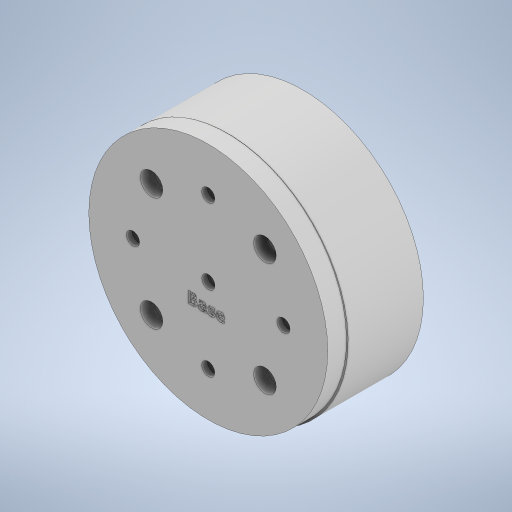
# Autodesk Inventor part: adaptor_spine_base_names
Saved by Autodesk Inventor 2024 (Build 280153000, 153)
## iProperties
Created: 2024-05-24
Part Number: adaptor_spine_base_names
Material: Generic
Document SubType Name: Modeling
Designer: maint
Density: 1 g/cm^3
Appearance: Default
Author: maint
Autodesk Inventor part; units mm, degrees
ref_plane "YZ Plane" through (0, 0, 0) normal (1, 0, 0) x (0, 1, 0)
ref_plane "XZ Plane" through (0, 0, 0) normal (0, 1, 0) x (-1, 0, 0)
ref_plane "XY Plane" through (0, 0, 0) normal (0, 0, 1) x (1, 0, 0)
sketch "Sketch1" plane through (0, 0, 0) normal (0, 0, 1) x (1, 0, 0)
  line L0 (40, -40) -> (-40, -40)
  line L1 (-40, -40) -> (-40, 40)
  line L2 (-40, 40) -> (40, 40)
  line L3 (40, 40) -> (40, -40)
  line L4 (40, -40) -> (-40, 40) construction
  line L5 (-40, -40) -> (40, 40) construction
  circle A0 centre (0, 0) radius 63.5
  dimension "d0" = 80
  dimension "d72" = 127
  constraints: 12 end point, 2 midpoint, 2 parallel, 2 perpendicular, 1 centre point, 1 coincident, 1 horizontal
  measures "d0" distance of L1.end L2.end
  measures "d72" diameter of A0
extrude "Extrusion1" add sketch "Sketch1" along normal blind 10 contours L0 L1 L2 L3 | A0
sketch "Sketch2" plane through (0, 0, 0) normal (0, 0, -1) x (-1, 0, 0)
  arc A0 (40, 37) -> (37, 40) centre (37, 37) ccw
  line L0 (30.15, -30.15) -> (-30.15, -30.15)
  line L1 (-30.15, -30.15) -> (-30.15, 30.15)
  line L2 (-30.15, 30.15) -> (30.15, 30.15)
  line L3 (30.15, 30.15) -> (30.15, -30.15)
  line L4 (30.15, -30.15) -> (-30.15, 30.15) construction
  line L5 (-30.15, -30.15) -> (30.15, 30.15) construction
  circle A1 centre (-30.15, 30.15) radius 4.75
  circle A2 centre (30.15, 30.15) radius 4.75
  circle A3 centre (30.15, -30.15) radius 4.75
  circle A4 centre (-30.15, -30.15) radius 4.75
  point P0 (0, 0)
  point P1 (39.1213, 39.1213)
  dimension "d32" = 60.3
  dimension "d33" = 9.5
  constraints: 12 end point, 5 centre point, 4 coincident, 3 equal radius, 3 point on circle, 2 midpoint, 2 parallel, 2 perpendicular, 1 horizontal
  measures "d32" distance of L1.end L2.end
  measures "d33" diameter of A2
hole "Hole3" at (30.15, -30.15, 0) at (30.15, 30.15, 0) at (-30.15, 30.15, 0) at (-30.15, -30.15, 0) direction (0, 0, 1) diameter 6.6 end through all
sketch "Sketch3" plane through (0, 0, 0) normal (0, 0, -1) x (-1, 0, 0)
  circle A0 centre (0, 0) radius 40
  circle A1 centre (0, 40) radius 2.5
  circle A2 centre (40, 0) radius 2.5
  circle A3 centre (0, -40) radius 2.5
  circle A4 centre (-40, 0) radius 2.5
  circle A5 centre (-0.0779, 0.0489) radius 2.5
  dimension "d12" = 5
  dimension "d60" = 80
  dimension "d74" = 5
  constraints: 6 centre point, 4 point on circle, 3 equal radius
  measures "d12" diameter of A1
  measures "d60" diameter of A0
  measures "d74" diameter of A5
hole "Hole1" at (40, 0, 0) at (0, 40, 0) at (0, -40, 0) at (-40, 0, 0) at (0.0779, 0.0489, 0) direction (0, 0, 1) diameter 7 end through all
sketch "Sketch8" plane through (0, 0, 0) normal (0, 0, -1) x (-1, 0, 0)
  circle A0 centre (0, 0) radius 40
  circle A1 centre (0, 40) radius 12.0233
  circle A2 centre (40, 0) radius 12.001
  circle A3 centre (-40, 0) radius 12.185
  circle A4 centre (0, -40) radius 12.001
  circle A5 centre (-0.3746, -0.3656) radius 12.0233
  dimension "d61" = 80
  constraints: 6 centre point, 4 point on circle
  measures "d61" diameter of A0
hole "Hole4" at (-40, 0, 0) at (0, 40, 0) at (40, 0, 0) at (0, -40, 0) at (0.3746, -0.3656, 0) direction (0, 0, 1) diameter 17 depth 7
sketch "Sketch10" plane through (0, 0, 10) normal (0, 0, 1) x (1, 0, 0)
  circle A0 centre (30.15, 30.15) radius 3.3 projected
  circle A1 centre (30.15, 30.15) radius 6
  circle A2 centre (-30.15, 30.15) radius 3.3 projected
  circle A3 centre (-30.15, 30.15) radius 6
  circle A4 centre (-30.15, -30.2444) radius 6
  circle A5 centre (30.15, -30.2444) radius 6
  point P0 (0, 0)
  dimension "d63" = 12
  constraints: 4 centre point, 3 equal radius, 2 coincident
  measures "d63" diameter of A1
hole "Hole5" at (-30.15, -30.2444, 10) at (30.15, -30.2444, 10) at (30.15, 30.15, 10) at (-30.15, 30.15, 10) direction (0, 0, -1) diameter 12 depth 7
sketch "Sketch11" plane through (-1.9817, 2.6504, 0) normal (0, 0, -1) x (-1, 0, 0)
  line L0 (-12.9782, -14.2221) -> (9.0418, -14.2221) construction
  line L1 (9.0418, -14.2221) -> (9.0418, -6.8756) construction
  line L2 (9.0418, -6.8756) -> (-12.9782, -6.8756) construction
  line L3 (-12.9782, -6.8756) -> (-12.9782, -14.2221) construction
  spline S0 degree 2 poles (-10.4621, -20.5396) (-11.164, -20.5396) (-12.2219, -20.2677) (-12.6767, -20.07) knots 0 0 0 1 2 2 2
  line L4 (-12.6767, -20.07) -> (-12.6767, -18.6166)
  line L5 (-12.6767, -18.6166) -> (-12.5383, -18.6166)
  spline S1 degree 2 poles (-12.5383, -18.6166) (-12.0785, -19.0072) (-10.9762, -19.4273) (-10.4571, -19.4273) knots 0 0 0 1 2 2 2
  spline S2 degree 2 poles (-10.4571, -19.4273) (-10.3237, -19.4273) (-9.8936, -19.368) (-9.7651, -19.3087) knots 0 0 0 1 2 2 2
  spline S3 degree 2 poles (-9.7651, -19.3087) (-9.6069, -19.2395) (-9.3845, -18.9874) (-9.3845, -18.7847) knots 0 0 0 1 2 2 2
  spline S4 degree 2 poles (-9.3845, -18.7847) (-9.3845, -18.5524) (-9.7453, -18.2657) (-9.9925, -18.2014) knots 0 0 0 1 2 2 2
  spline S5 degree 2 poles (-9.9925, -18.2014) (-10.3039, -18.1174) (-11.0108, -17.974) (-11.3222, -17.8653) knots 0 0 0 1 2 2 2
  spline S6 degree 2 poles (-11.3222, -17.8653) (-12.0291, -17.6181) (-12.6421, -16.7728) (-12.6421, -16.1401) knots 0 0 0 1 2 2 2
  spline S7 degree 2 poles (-12.6421, -16.1401) (-12.6421, -15.2849) (-11.1937, -14.2221) (-10.1062, -14.2221) knots 0 0 0 1 2 2 2
  spline S8 degree 2 poles (-10.1062, -14.2221) (-9.5624, -14.2221) (-8.4848, -14.4445) (-8.0597, -14.6324) knots 0 0 0 1 2 2 2
  line L6 (-8.0597, -14.6324) -> (-8.0597, -16.0264)
  line L7 (-8.0597, -16.0264) -> (-8.1931, -16.0264)
  spline S9 degree 2 poles (-8.1931, -16.0264) (-8.5342, -15.7347) (-9.513, -15.3343) (-10.0271, -15.3343) knots 0 0 0 1 2 2 2
  spline S10 degree 2 poles (-10.0271, -15.3343) (-10.2298, -15.3343) (-10.5461, -15.3936) (-10.7241, -15.4727) knots 0 0 0 1 2 2 2
  spline S11 degree 2 poles (-10.7241, -15.4727) (-10.8674, -15.537) (-11.0751, -15.794) (-11.0751, -15.9522) knots 0 0 0 1 2 2 2
  spline S12 degree 2 poles (-11.0751, -15.9522) (-11.0751, -16.1895) (-10.7439, -16.4614) (-10.2693, -16.5701) knots 0 0 0 1 2 2 2
  spline S13 degree 2 poles (-10.2693, -16.5701) (-9.9628, -16.6393) (-9.3943, -16.7728) (-9.0681, -16.8865) knots 0 0 0 1 2 2 2
  spline S14 degree 2 poles (-9.0681, -16.8865) (-8.4353, -17.1188) (-7.8174, -17.89) (-7.8174, -18.5227) knots 0 0 0 1 2 2 2
  spline S15 degree 2 poles (-7.8174, -18.5227) (-7.8174, -19.4323) (-9.246, -20.5396) (-10.4621, -20.5396) knots 0 0 0 1 2 2 2
  spline S16 degree 2 poles (-2.3403, -16.2538) (-2.3403, -16.6789) (-2.6122, -17.45) (-2.8643, -17.7071) knots 0 0 0 1 2 2 2
  spline S17 degree 2 poles (-2.8643, -17.7071) (-3.0175, -17.8702) (-3.3932, -18.1371) (-3.6157, -18.2311) knots 0 0 0 1 2 2 2
  spline S18 degree 2 poles (-3.6157, -18.2311) (-3.843, -18.325) (-4.372, -18.4337) (-4.6982, -18.4337) knots 0 0 0 1 2 2 2
  line L8 (-4.6982, -18.4337) -> (-5.499, -18.4337)
  line L9 (-5.499, -18.4337) -> (-5.499, -20.4308)
  line L10 (-5.499, -20.4308) -> (-7.0315, -20.4308)
  line L11 (-7.0315, -20.4308) -> (-7.0315, -14.3308)
  line L12 (-7.0315, -14.3308) -> (-4.6636, -14.3308)
  spline S19 degree 2 poles (-4.6636, -14.3308) (-4.1396, -14.3308) (-3.3734, -14.5236) (-3.062, -14.7312) knots 0 0 0 1 2 2 2
  spline S20 degree 2 poles (-3.062, -14.7312) (-2.716, -14.9636) (-2.3403, -15.7248) (-2.3403, -16.2538) knots 0 0 0 1 2 2 2
  spline S21 degree 2 poles (-3.9122, -16.2933) (-3.9122, -16.0313) (-4.1594, -15.6606) (-4.3275, -15.5914) knots 0 0 0 1 2 2 2
  spline S22 degree 2 poles (-4.3275, -15.5914) (-4.545, -15.4974) (-4.9404, -15.4678) (-5.2815, -15.4678) knots 0 0 0 1 2 2 2
  line L13 (-5.2815, -15.4678) -> (-5.499, -15.4678)
  line L14 (-5.499, -15.4678) -> (-5.499, -17.2968)
  line L15 (-5.499, -17.2968) -> (-5.3903, -17.2968)
  spline S23 degree 2 poles (-5.3903, -17.2968) (-5.1777, -17.2968) (-4.7922, -17.2869) (-4.6488, -17.2622) knots 0 0 0 1 2 2 2
  spline S24 degree 2 poles (-4.6488, -17.2622) (-4.5252, -17.2424) (-4.2533, -17.1238) (-4.1792, -17.0496) knots 0 0 0 1 2 2 2
  spline S25 degree 2 poles (-4.1792, -17.0496) (-4.021, -16.9013) (-3.9122, -16.5701) (-3.9122, -16.2933) knots 0 0 0 1 2 2 2
  line L16 (1.5155, -20.4308) -> (-1.7669, -20.4308)
  line L17 (-1.7669, -20.4308) -> (-1.7669, -19.368)
  line L18 (-1.7669, -19.368) -> (-0.8919, -19.368)
  line L19 (-0.8919, -19.368) -> (-0.8919, -15.3936)
  line L20 (-0.8919, -15.3936) -> (-1.7669, -15.3936)
  line L21 (-1.7669, -15.3936) -> (-1.7669, -14.3308)
  line L22 (-1.7669, -14.3308) -> (1.5155, -14.3308)
  line L23 (1.5155, -14.3308) -> (1.5155, -15.3936)
  line L24 (1.5155, -15.3936) -> (0.6405, -15.3936)
  line L25 (0.6405, -15.3936) -> (0.6405, -19.368)
  line L26 (0.6405, -19.368) -> (1.5155, -19.368)
  line L27 (1.5155, -19.368) -> (1.5155, -20.4308)
  line L28 (7.7588, -20.4308) -> (6.2857, -20.4308)
  line L29 (6.2857, -20.4308) -> (3.9327, -16.1796)
  line L30 (3.9327, -16.1796) -> (3.9327, -20.4308)
  line L31 (3.9327, -20.4308) -> (2.5338, -20.4308)
  line L32 (2.5338, -20.4308) -> (2.5338, -14.3308)
  line L33 (2.5338, -14.3308) -> (4.4122, -14.3308)
  line L34 (4.4122, -14.3308) -> (6.3599, -17.8257)
  line L35 (6.3599, -17.8257) -> (6.3599, -14.3308)
  line L36 (6.3599, -14.3308) -> (7.7588, -14.3308)
  line L37 (7.7588, -14.3308) -> (7.7588, -20.4308)
  line L38 (8.9996, -20.4308) -> (8.9996, -14.3308)
  line L39 (8.9996, -14.3308) -> (13.1223, -14.3308)
  line L40 (13.1223, -14.3308) -> (13.1223, -15.4925)
  line L41 (13.1223, -15.4925) -> (10.5221, -15.4925)
  line L42 (10.5221, -15.4925) -> (10.5221, -16.5652)
  line L43 (10.5221, -16.5652) -> (12.9196, -16.5652)
  line L44 (12.9196, -16.5652) -> (12.9196, -17.7268)
  line L45 (12.9196, -17.7268) -> (10.5221, -17.7268)
  line L46 (10.5221, -17.7268) -> (10.5221, -19.2692)
  line L47 (10.5221, -19.2692) -> (13.1223, -19.2692)
  line L48 (13.1223, -19.2692) -> (13.1223, -20.4308)
  line L49 (13.1223, -20.4308) -> (8.9996, -20.4308)
  point P0 (0, 0)
  constraints: 2 other
extrude "Extrusion5" cut sketch "Sketch11" against normal blind 1
sketch "Sketch12" plane through (-4.4722, 1.3995, 10) normal (0, 0, 1) x (1, 0, 0)
  line L0 (-6.7643, -10.3972) -> (19.0988, -10.3972) construction
  line L1 (19.0988, -10.3972) -> (19.0988, -6.1489) construction
  line L2 (19.0988, -6.1489) -> (-6.7643, -6.1489) construction
  line L3 (-6.7643, -6.1489) -> (-6.7643, -10.3972) construction
  spline S0 degree 2 poles (-1.2575, -14.6287) (-1.2575, -15.0834) (-1.6035, -15.7705) (-1.8902, -15.9979) knots 0 0 0 1 2 2 2
  spline S1 degree 2 poles (-1.8902, -15.9979) (-2.2362, -16.2698) (-3.0568, -16.4972) (-3.6945, -16.4972) knots 0 0 0 1 2 2 2
  line L4 (-3.6945, -16.4972) -> (-6.1315, -16.4972)
  line L5 (-6.1315, -16.4972) -> (-6.1315, -10.3972)
  line L6 (-6.1315, -10.3972) -> (-3.9812, -10.3972)
  spline S2 degree 2 poles (-3.9812, -10.3972) (-3.3089, -10.3972) (-2.6169, -10.501) (-2.3153, -10.6641) knots 0 0 0 1 2 2 2
  spline S3 degree 2 poles (-2.3153, -10.6641) (-1.9841, -10.8372) (-1.6628, -11.4304) (-1.6628, -11.8159) knots 0 0 0 1 2 2 2
  spline S4 degree 2 poles (-1.6628, -11.8159) (-1.6628, -12.2608) (-2.1077, -12.9578) (-2.5032, -13.121) knots 0 0 0 1 2 2 2
  line L7 (-2.5032, -13.121) -> (-2.5032, -13.1506)
  spline S5 degree 2 poles (-2.5032, -13.1506) (-1.9347, -13.2693) (-1.2575, -14.0058) (-1.2575, -14.6287) knots 0 0 0 1 2 2 2
  spline S6 degree 2 poles (-2.8393, -14.6039) (-2.8393, -14.3172) (-3.0667, -13.9959) (-3.2941, -13.9119) knots 0 0 0 1 2 2 2
  spline S7 degree 2 poles (-3.2941, -13.9119) (-3.4325, -13.8575) (-3.9219, -13.8476) (-4.3272, -13.8476) knots 0 0 0 1 2 2 2
  line L8 (-4.3272, -13.8476) -> (-4.609, -13.8476)
  line L9 (-4.609, -13.8476) -> (-4.609, -15.385)
  line L10 (-4.609, -15.385) -> (-4.525, -15.385)
  spline S8 degree 2 poles (-4.525, -15.385) (-3.9318, -15.385) (-3.477, -15.3701) (-3.2397, -15.2663) knots 0 0 0 1 2 2 2
  spline S9 degree 2 poles (-3.2397, -15.2663) (-3.0321, -15.1724) (-2.8393, -14.8264) (-2.8393, -14.6039) knots 0 0 0 1 2 2 2
  spline S10 degree 2 poles (-3.2199, -12.1175) (-3.2199, -11.9692) (-3.3732, -11.6577) (-3.5314, -11.5885) knots 0 0 0 1 2 2 2
  spline S11 degree 2 poles (-3.5314, -11.5885) (-3.6797, -11.5193) (-4.0949, -11.5094) (-4.5052, -11.5094) knots 0 0 0 1 2 2 2
  line L11 (-4.5052, -11.5094) -> (-4.609, -11.5094)
  line L12 (-4.609, -11.5094) -> (-4.609, -12.8046)
  line L13 (-4.609, -12.8046) -> (-4.4162, -12.8046)
  spline S12 degree 2 poles (-4.4162, -12.8046) (-4.0257, -12.8046) (-3.7093, -12.7898) (-3.5412, -12.7107) knots 0 0 0 1 2 2 2
  spline S13 degree 2 poles (-3.5412, -12.7107) (-3.3583, -12.6217) (-3.2199, -12.3201) (-3.2199, -12.1175) knots 0 0 0 1 2 2 2
  spline S14 degree 2 poles (2.0743, -16.0078) (1.926, -16.1314) (1.6937, -16.3291) (1.496, -16.428) knots 0 0 0 1 2 2 2
  spline S15 degree 2 poles (1.496, -16.428) (1.3032, -16.5219) (0.9374, -16.6208) (0.6111, -16.6208) knots 0 0 0 1 2 2 2
  spline S16 degree 2 poles (0.6111, -16.6208) (-0.0019, -16.6208) (-0.8076, -15.8002) (-0.8076, -15.1774) knots 0 0 0 1 2 2 2
  spline S17 degree 2 poles (-0.8076, -15.1774) (-0.8076, -14.6682) (-0.3973, -14.0355) (-0.0117, -13.8526) knots 0 0 0 1 2 2 2
  spline S18 degree 2 poles (-0.0117, -13.8526) (0.3788, -13.6647) (1.4613, -13.5164) (2.0842, -13.4769) knots 0 0 0 1 2 2 2
  line L14 (2.0842, -13.4769) -> (2.0842, -13.4522)
  spline S19 degree 2 poles (2.0842, -13.4522) (2.0842, -13.0715) (1.5207, -12.7799) (0.9571, -12.7799) knots 0 0 0 1 2 2 2
  spline S20 degree 2 poles (0.9571, -12.7799) (0.705, -12.7799) (0.0229, -12.9628) (-0.2985, -13.1061) knots 0 0 0 1 2 2 2
  line L15 (-0.2985, -13.1061) -> (-0.422, -13.1061)
  line L16 (-0.422, -13.1061) -> (-0.422, -11.9939)
  spline S21 degree 2 poles (-0.422, -11.9939) (-0.2095, -11.9346) (0.7396, -11.7665) (1.2241, -11.7665) knots 0 0 0 1 2 2 2
  spline S22 degree 2 poles (1.2241, -11.7665) (2.4105, -11.7665) (3.498, -12.5574) (3.498, -13.3681) knots 0 0 0 1 2 2 2
  line L17 (3.498, -13.3681) -> (3.498, -16.4972)
  line L18 (3.498, -16.4972) -> (2.0743, -16.4972)
  line L19 (2.0743, -16.4972) -> (2.0743, -16.0078)
  line L20 (2.0743, -15.296) -> (2.0743, -14.3419)
  spline S23 degree 2 poles (2.0743, -14.3419) (1.7085, -14.3765) (1.2587, -14.4309) (1.0412, -14.51) knots 0 0 0 1 2 2 2
  spline S24 degree 2 poles (1.0412, -14.51) (0.8484, -14.5743) (0.6408, -14.8412) (0.6408, -15.0587) knots 0 0 0 1 2 2 2
  spline S25 degree 2 poles (0.6408, -15.0587) (0.6408, -15.38) (0.9917, -15.6223) (1.3328, -15.6223) knots 0 0 0 1 2 2 2
  spline S26 degree 2 poles (1.3328, -15.6223) (1.5207, -15.6223) (1.9161, -15.4492) (2.0743, -15.296) knots 0 0 0 1 2 2 2
  spline S27 degree 2 poles (5.9597, -16.6208) (5.4555, -16.6208) (4.5509, -16.3983) (4.2543, -16.25) knots 0 0 0 1 2 2 2
  line L21 (4.2543, -16.25) -> (4.2543, -15.0389)
  line L22 (4.2543, -15.0389) -> (4.3729, -15.0389)
  spline S28 degree 2 poles (4.3729, -15.0389) (4.4767, -15.118) (4.7387, -15.3059) (4.9711, -15.4097) knots 0 0 0 1 2 2 2
  spline S29 degree 2 poles (4.9711, -15.4097) (5.1737, -15.5036) (5.673, -15.6371) (5.9696, -15.6371) knots 0 0 0 1 2 2 2
  spline S30 degree 2 poles (5.9696, -15.6371) (6.2712, -15.6371) (6.7358, -15.4492) (6.7358, -15.2466) knots 0 0 0 1 2 2 2
  spline S31 degree 2 poles (6.7358, -15.2466) (6.7358, -15.0884) (6.5233, -14.9203) (6.2168, -14.8511) knots 0 0 0 1 2 2 2
  spline S32 degree 2 poles (6.2168, -14.8511) (6.0536, -14.8066) (5.5544, -14.7127) (5.3616, -14.6534) knots 0 0 0 1 2 2 2
  spline S33 degree 2 poles (5.3616, -14.6534) (4.8178, -14.4853) (4.2741, -13.8278) (4.2741, -13.289) knots 0 0 0 1 2 2 2
  spline S34 degree 2 poles (4.2741, -13.289) (4.2741, -12.9825) (4.5558, -12.4388) (4.8327, -12.2262) knots 0 0 0 1 2 2 2
  spline S35 degree 2 poles (4.8327, -12.2262) (5.1045, -12.0186) (5.9103, -11.7714) (6.4195, -11.7714) knots 0 0 0 1 2 2 2
  spline S36 degree 2 poles (6.4195, -11.7714) (6.9039, -11.7714) (7.7146, -11.9642) (7.9914, -12.0977) knots 0 0 0 1 2 2 2
  line L23 (7.9914, -12.0977) -> (7.9914, -13.2643)
  line L24 (7.9914, -13.2643) -> (7.8777, -13.2643)
  spline S37 degree 2 poles (7.8777, -13.2643) (7.8036, -13.205) (7.4823, -13.0122) (7.334, -12.943) knots 0 0 0 1 2 2 2
  spline S38 degree 2 poles (7.334, -12.943) (7.1511, -12.8639) (6.7062, -12.7552) (6.4738, -12.7552) knots 0 0 0 1 2 2 2
  spline S39 degree 2 poles (6.4738, -12.7552) (6.1624, -12.7552) (5.7323, -12.9677) (5.7323, -13.1407) knots 0 0 0 1 2 2 2
  spline S40 degree 2 poles (5.7323, -13.1407) (5.7323, -13.2989) (5.9449, -13.4769) (6.3008, -13.5658) knots 0 0 0 1 2 2 2
  spline S41 degree 2 poles (6.3008, -13.5658) (6.4837, -13.6103) (6.9632, -13.6944) (7.1857, -13.7685) knots 0 0 0 1 2 2 2
  spline S42 degree 2 poles (7.1857, -13.7685) (7.68, -13.9267) (8.1941, -14.5446) (8.1941, -15.0587) knots 0 0 0 1 2 2 2
  spline S43 degree 2 poles (8.1941, -15.0587) (8.1941, -15.38) (7.8925, -15.9683) (7.6108, -16.166) knots 0 0 0 1 2 2 2
  spline S44 degree 2 poles (7.6108, -16.166) (7.3191, -16.3835) (6.5183, -16.6208) (5.9597, -16.6208) knots 0 0 0 1 2 2 2
  spline S45 degree 2 poles (11.2342, -16.6208) (9.9292, -16.6208) (8.5401, -15.3751) (8.5401, -14.2233) knots 0 0 0 1 2 2 2
  spline S46 degree 2 poles (8.5401, -14.2233) (8.5401, -13.0962) (9.8353, -11.7517) (11.0019, -11.7517) knots 0 0 0 1 2 2 2
  spline S47 degree 2 poles (11.0019, -11.7517) (12.0548, -11.7517) (13.1225, -12.8936) (13.1225, -13.9514) knots 0 0 0 1 2 2 2
  line L25 (13.1225, -13.9514) -> (13.1225, -14.4705)
  line L26 (13.1225, -14.4705) -> (9.9737, -14.4705)
  spline S48 degree 2 poles (9.9737, -14.4705) (9.9934, -14.7918) (10.2258, -15.2169) (10.4136, -15.3454) knots 0 0 0 1 2 2 2
  spline S49 degree 2 poles (10.4136, -15.3454) (10.5965, -15.474) (11.0908, -15.5827) (11.3825, -15.5827) knots 0 0 0 1 2 2 2
  spline S50 degree 2 poles (11.3825, -15.5827) (11.6297, -15.5827) (12.1141, -15.474) (12.3168, -15.38) knots 0 0 0 1 2 2 2
  spline S51 degree 2 poles (12.3168, -15.38) (12.4947, -15.3059) (12.7913, -15.123) (12.8853, -15.0538) knots 0 0 0 1 2 2 2
  line L27 (12.8853, -15.0538) -> (13.0385, -15.0538)
  line L28 (13.0385, -15.0538) -> (13.0385, -16.2402)
  spline S52 degree 2 poles (13.0385, -16.2402) (12.8605, -16.3094) (12.5738, -16.428) (12.3168, -16.4873) knots 0 0 0 1 2 2 2
  spline S53 degree 2 poles (12.3168, -16.4873) (12.0844, -16.5516) (11.5901, -16.6208) (11.2342, -16.6208) knots 0 0 0 1 2 2 2
  spline S54 degree 2 poles (11.7088, -13.6054) (11.6989, -13.1506) (11.2985, -12.6711) (10.8882, -12.6711) knots 0 0 0 1 2 2 2
  spline S55 degree 2 poles (10.8882, -12.6711) (10.468, -12.6711) (9.9934, -13.1753) (9.9687, -13.6054) knots 0 0 0 1 2 2 2
  line L29 (9.9687, -13.6054) -> (11.7088, -13.6054)
  point P0 (0, 0)
  constraints: 2 other
extrude "Extrusion6" cut sketch "Sketch12" against normal blind 1
sketch "Sketch13" plane through (-11.7041, 34.1674, 0) normal (0, 0, -1) x (-1, 0, 0)
  line L0 (-1.7664, -61.241) -> (-17.5943, -76.9041) construction
  line L1 (-17.5943, -76.9041) -> (-22.3671, -72.081) construction
  line L2 (-22.3671, -72.081) -> (-6.5391, -56.4179) construction
  line L3 (-6.5391, -56.4179) -> (-1.7664, -61.241) construction
  line L4 (-5.7167, -57.8268) -> (-9.8926, -61.9592) construction
  line L5 (-9.8926, -61.9592) -> (-35.8899, -35.6882) construction
  line L6 (-35.8899, -35.6882) -> (-31.714, -31.5558) construction
  line L7 (-31.714, -31.5558) -> (-5.7167, -57.8268) construction
  line L8 (-5.3015, -58.7064) -> (-0.2981, -58.7064) construction
  line L9 (-0.2981, -58.7064) -> (-0.2981, -61.8764) construction
  line L10 (-0.2981, -61.8764) -> (-5.3015, -61.8764) construction
  line L11 (-5.3015, -61.8764) -> (-5.3015, -58.7064) construction
  line L12 (-17.522, -55.7631) -> (-14.084, -55.7631) construction
  line L13 (-14.084, -55.7631) -> (-14.084, -61.3066) construction
  line L14 (-14.084, -61.3066) -> (-17.522, -61.3066) construction
  line L15 (-17.522, -61.3066) -> (-17.522, -55.7631) construction
  line L16 (-7.756, -62.0484) -> (-6.5724, -62.0437)
  line L17 (-6.5724, -62.0437) -> (-6.5566, -57.4699)
  line L18 (-6.5566, -57.4699) -> (-6.0327, -57.4591)
  line L19 (-6.0327, -57.4591) -> (-6.0594, -62.0437)
  line L20 (-6.0594, -62.0437) -> (-4.8922, -62.0552)
  line L21 (-4.8922, -62.0552) -> (-6.3372, -65.8452)
  line L22 (-6.3372, -65.8452) -> (-7.756, -62.0484)
  line L23 (-10.7, -55.9696) -> (-10.6954, -57.1531)
  line L24 (-10.6954, -57.1531) -> (-6.1216, -57.1689)
  line L25 (-6.1216, -57.1689) -> (-6.1107, -57.6929)
  line L26 (-6.1107, -57.6929) -> (-10.6953, -57.6661)
  line L27 (-10.6953, -57.6661) -> (-10.7069, -58.8333)
  line L28 (-10.7069, -58.8333) -> (-14.4968, -57.3884)
  line L29 (-14.4968, -57.3884) -> (-10.7, -55.9696)
  line L30 (-14.5113, -58.9331) -> (-15.4309, -58.9331)
  line L31 (-15.4309, -58.9331) -> (-16.0423, -57.9235)
  line L32 (-16.0423, -57.9235) -> (-16.6666, -58.9331)
  line L33 (-16.6666, -58.9331) -> (-17.5477, -58.9331)
  line L34 (-17.5477, -58.9331) -> (-16.5176, -57.3378)
  line L35 (-16.5176, -57.3378) -> (-17.5066, -55.7631)
  line L36 (-17.5066, -55.7631) -> (-16.5869, -55.7631)
  line L37 (-16.5869, -55.7631) -> (-16.0141, -56.7213)
  line L38 (-16.0141, -56.7213) -> (-15.4258, -55.7631)
  line L39 (-15.4258, -55.7631) -> (-14.5447, -55.7631)
  line L40 (-14.5447, -55.7631) -> (-15.5388, -57.3044)
  line L41 (-15.5388, -57.3044) -> (-14.5113, -58.9331)
  line L42 (-2.337, -58.7064) -> (-3.4313, -60.5534)
  line L43 (-3.4313, -60.5534) -> (-3.4313, -61.8764)
  line L44 (-3.4313, -61.8764) -> (-4.2277, -61.8764)
  line L45 (-4.2277, -61.8764) -> (-4.2277, -60.592)
  line L46 (-4.2277, -60.592) -> (-5.34, -58.7064)
  line L47 (-5.34, -58.7064) -> (-4.4332, -58.7064)
  line L48 (-4.4332, -58.7064) -> (-3.8141, -59.8367)
  line L49 (-3.8141, -59.8367) -> (-3.2155, -58.7064)
  line L50 (-3.2155, -58.7064) -> (-2.337, -58.7064)
  point P0 (0, 0)
  constraints: 8 other
extrude "Extrusion7" cut sketch "Sketch13" against normal blind 1
sketch "Sketch14" plane through (0, 0, 0) normal (0, 0, -1) x (-1, 0, 0)
  circle A0 centre (-0.0779, 0.0489) radius 3.5 projected
  circle A1 centre (-0.0779, 0.0489) radius 55
  circle A2 centre (-0.3746, -0.3656) radius 8.5 projected
  circle A3 centre (-0.3746, -0.3656) radius 63.9792
  point P0 (0, 0)
  dimension "d84" = 110
  constraints: 2 centre point, 2 coincident
  measures "d84" diameter of A1
extrude "Extrusion8" add sketch "Sketch14" along normal blind 40 contours A3
body "Solid1"
